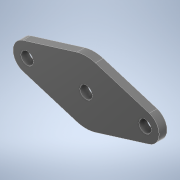
# Autodesk Inventor part: Pison Shaft Replacement Screw Plate
Saved by Autodesk Inventor 2021 (Build 250183000, 183)
## iProperties
Created: 2021-03-25
Part Number: Pison Shaft Replacement Screw Plate
Material: Thermoplastic Resin
Document SubType Name: Modeling
Designer: aidan
Density: 1.28 g/cm^3
Appearance: Smooth - Black
Author: aidan
Autodesk Inventor part; units mm, degrees
ref_plane "YZ Plane" through (0, 0, 0) normal (1, 0, 0) x (0, 1, 0)
ref_plane "XZ Plane" through (0, 0, 0) normal (0, 1, 0) x (-1, 0, 0)
ref_plane "XY Plane" through (0, 0, 0) normal (0, 0, 1) x (1, 0, 0)
sketch "Sketch1" plane through (0, 0, 0) normal (0, 0, 1) x (1, 0, 0)
  circle A0 centre (0, 0) radius 23.8125 construction
  circle A1 centre (-23.8125, 0) radius 2.4892
  circle A2 centre (23.8125, 0) radius 2.4892
  line L0 (-23.8125, 0) -> (23.8125, 0) construction
  circle A3 centre (0, 0) radius 2.4892
  arc A4 (-25.4861, 5.4113) -> (-25.4861, -5.4113) centre (-23.8125, 0) ccw
  arc A5 (25.4861, -5.4113) -> (25.4861, 5.4113) centre (23.8125, 0) ccw
  line L1 (-25.4861, 5.4113) -> (-3.7524, 12.133)
  line L2 (3.7524, 12.133) -> (25.4861, 5.4113)
  line L3 (25.4861, -5.4113) -> (3.7524, -12.133)
  line L4 (-3.7524, -12.133) -> (-25.4861, -5.4113)
  arc A6 (-3.7524, -12.133) -> (3.7524, -12.133) centre (0, 0) ccw
  arc A7 (3.7524, 12.133) -> (-3.7524, 12.133) centre (0, 0) ccw
  dimension "d0" = 47.625
  dimension "d1" = 4.9784
  dimension "d2" = 3.175
  dimension "d4" = 12.7
  dimension "d5" = 12.7
  constraints: 10 end point, 10 point on circle, 8 centre point, 8 tangent, 5 coincident, 3 equal radius, 1 horizontal, 1 midpoint
  measures "d0" diameter of A0
  measures "d1" diameter of A1
  measures "d2" radial gap between concentric circles of A1 A4
  measures "d4" radius of A7
  measures "d5" radius of A6
extrude "Extrusion1" add sketch "Sketch1" along normal blind 3.175
body "Solid1"
